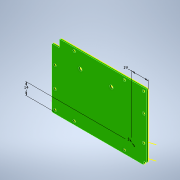
# Autodesk Inventor part: TCU_UCU_PCB
Saved by Autodesk Inventor 2021 (Build 250183000, 183)
## iProperties
Created: 2020-02-26
Part Number: TCU_UCU_PCB
Material: Generic
Document SubType Name: Modeling
Designer: lgnds
Density: 1 g/cm^3
Appearance: Default
Author: lgnds
Autodesk Inventor part; units mm, degrees
ref_plane "YZ Plane" through (0, 0, 0) normal (1, 0, 0) x (0, 1, 0)
ref_plane "XZ Plane" through (0, 0, 0) normal (0, 1, 0) x (-1, 0, 0)
ref_plane "XY Plane" through (0, 0, 0) normal (0, 0, 1) x (1, 0, 0)
sketch "Sketch1" plane through (0, 0, 0) normal (0, 0, 1) x (1, 0, 0)
  line L0 (-56.1965, -39.8485) -> (56.1965, -39.8485)
  line L1 (56.1965, -39.8485) -> (56.1965, 39.8485)
  line L2 (56.1965, 39.8485) -> (-56.1965, 39.8485)
  line L3 (-56.1965, 39.8485) -> (-56.1965, -39.8485)
  line L4 (-56.1965, -39.8485) -> (56.1965, 39.8485) construction
  line L5 (56.1965, -39.8485) -> (-56.1965, 39.8485) construction
  point P0 (0, 0)
  dimension "d0" = 79.697
  dimension "d1" = 112.393
  constraints: 12 end point, 2 midpoint, 2 parallel, 1 horizontal, 1 perpendicular
  measures "d0" distance of L2.end L0.start
  measures "d1" distance of L1.end L2.end
extrude "Extrusion1" add sketch "Sketch1" along normal blind 1.6
sketch "Sketch2" plane through (0, 0, 1.6) normal (0, 0, 1) x (1, 0, 0)
  line L0 (0, 0) -> (-76.7169, 0) construction
  line L1 (-76.7169, 0) -> (-68.8856, 0) construction
  line L2 (-56.1965, 39.8485) -> (-56.1965, -39.8485) construction
  circle A0 centre (-51.6965, 12.8485) radius 1.6
  line L3 (0, 55.7879) -> (0, -55.7879) construction
  line L4 (76.7169, 0) -> (68.8856, 0) construction
  line L5 (56.1965, 39.8485) -> (-56.1965, 39.8485) projected
  line L6 (-78.3509, -2) -> (74.4139, -2) construction
  line L7 (56.1965, 39.8485) -> (56.1965, -39.8485) construction
  circle A1 centre (51.6965, 12.8485) radius 1.6
  circle A2 centre (-51.6965, -16.8485) radius 1.6
  circle A3 centre (51.6965, -16.8485) radius 1.6
  dimension "d5" = 3.2
  dimension "d20" = 27
  dimension "d21" = 4.5
  dimension "d22" = 14.8485
  constraints: 10 end point, 6 symmetric about line, 4 centre point, 2 horizontal, 3 other
  measures "d5" diameter of A0
  measures "d20" distance from line of L5 A0.centre
  measures "d21" distance from line of L2 A0.centre
  measures "d22" distance from line of A0.centre L6
extrude "Extrusion2" cut sketch "Sketch2" against normal up to next
sketch "Sketch6" plane through (0, 0, 1.6) normal (0, 0, 1) x (1, 0, 0)
  line L0 (-64.772, 35.3485) -> (88.7849, 35.3485) construction
  circle A0 centre (-29.1965, 35.3485) radius 1.6
  line L1 (0, -55.7879) -> (0, 55.7879) construction
  line L2 (56.1965, 39.8485) -> (-56.1965, 39.8485) construction
  circle A1 centre (-51.6965, 12.8485) radius 1.6 projected
  line L3 (-95.4834, 0) -> (119.4963, 0) construction
  circle A2 centre (29.1965, 35.3485) radius 1.6
  circle A3 centre (-29.1965, -35.3485) radius 1.6
  circle A4 centre (29.1965, -35.3485) radius 1.6
  line L4 (-56.1965, 39.8485) -> (-56.1965, -39.8485) projected
  point P0 (0, 0)
  point P1 (-64.772, -35.3485)
  dimension "d23" = 3.2
  dimension "d24" = 4.5
  dimension "d36" = 27
  constraints: 4 centre point, 4 symmetric about line, 2 end point, 1 horizontal, 1 point on line, 3 other
  measures "d23" diameter of A0
  measures "d24" distance between parallel lines of L2 L0
  measures "d36" distance from line of L4 A0.centre
extrude "Extrusion5" cut sketch "Sketch6" against normal up to next contours A0 | A2 | A3 | A4
sketch "Sketch7" plane through (0, 0, 0) normal (0, 0, -1) x (-1, 0, 0)
  circle A0 centre (-14.1318, 20.7641) radius 1.9985
  arc A1 (51.6966, 24.8485) -> (51.6966, 14.8485) centre (51.6966, 19.8485) ccw
  line L0 (51.6966, 24.8485) -> (56.1965, 24.8485)
  line L1 (56.1965, 39.8485) -> (56.1965, -39.8485) construction
  line L2 (51.6966, 14.8485) -> (56.1965, 14.8485)
  line L3 (56.1965, 24.8485) -> (56.1965, 14.8485)
  circle A2 centre (22.0882, 20.7641) radius 1.9985
  line L4 (-91.8718, 0) -> (99.9198, 0) construction
  line L5 (-61.1962, -2.1515) -> (72.521, -2.1515) construction
  circle A3 centre (51.6966, -24.1515) radius 2 construction
  arc A4 (51.6966, -19.1515) -> (51.6966, -29.1515) centre (51.6966, -24.1515) ccw
  line L6 (51.6966, -29.1515) -> (56.1965, -29.1515)
  line L7 (56.1965, -44.1515) -> (56.1965, 35.5455) construction
  line L8 (51.6966, -19.1515) -> (56.1965, -19.1515)
  line L9 (56.1965, -29.1515) -> (56.1965, -19.1515)
  circle A5 centre (-14.1318, 20.7641) radius 1.4985 projected
  circle A6 centre (22.0882, 20.7641) radius 1.4985 projected
  circle A7 centre (51.6966, -24.1515) radius 2 projected
  circle A8 centre (51.6966, 19.8485) radius 2 projected
  point P0 (0, 0)
  dimension "d28" = 10
  dimension "d33" = 22
  constraints: 16 end point, 7 symmetric about line, 5 centre point, 4 point on circle, 4 point on line, 2 parallel, 2 tangent, 1 coincident, 1 horizontal, 2 other
  measures "d28" diameter of A1
  measures "d33" distance from line of A1.centre L5
extrude "Extrusion6" cut sketch "Sketch7" against normal up to next contours A0 | L0 L3 L2 A1 | A2 | L8 L9 L6 A4 | A5 | A6 | A7 | A8
thicken "Thicken1" operation add thickness 0.75 both sides no extend neighbours yes toward (-1, 0, 0) faces at (56.1965, -13.2828, 0.5333) (-18.7322, -39.8485, 0.5333) (-56.1965, -32.7172, 0.5333) (18.7322, 39.8485, 0.5333) (-56.1965, 34.8485, 0.5333)
thicken "Thicken2" operation add thickness 0.75 both sides no extend neighbours yes toward (1, 0, 0) faces at (-56.1965, 3.5152, 1.0667)
sketch "Sketch9" plane through (0, 0, 0) normal (0, 0, -1) x (-1, 0, 0)
  line L0 (-29.4046, -25) -> (-55.4465, -25)
  line L1 (-55.4465, -39.0985) -> (-55.4465, 39.0985) projected
  line L2 (55.4465, -39.0985) -> (-55.4465, -39.0985) projected
  line L3 (-42.5, -39.0985) -> (-42.5, -4.682)
  point P0 (0, 0)
  dimension "d43" = 42.5
  dimension "d44" = 25
  constraints: 4 end point, 2 point on line, 1 horizontal, 1 perpendicular
  measures "d43" distance from line of point (0, 0) L3
  measures "d44" distance from line of point (0, 0) L0
fillet "Fillet1" radius 1 6 edges at (-55.4465, -39.0985, 0.8) (-55.4465, -29.1515, 0.8) (-55.4465, -19.1515, 0.8) (55.4465, 39.0985, 0.8) (-55.4465, 24.8485, 0.8) (-55.4465, 14.8485, 0.8)
sketch "Sketch10" plane through (0, 0, 0) normal (0, 0, -1) x (-1, 0, 0)
  line L0 (55.4465, 39.0985) -> (46.4465, 39.0985)
  line L1 (46.4465, 39.0985) -> (46.4465, 30.0985)
  line L2 (46.4465, 30.0985) -> (55.4465, 30.0985)
  line L3 (55.4465, 30.0985) -> (55.4465, 39.0985)
  line L4 (-55.4465, -39.0985) -> (-55.4465, 38.0985) projected
  line L5 (-55.4465, -39.0985) -> (-51.6965, -39.0985)
  line L6 (-51.6965, -39.0985) -> (-51.6965, -35.3485)
  line L7 (-51.6965, -35.3485) -> (-55.4465, -35.3485)
  line L8 (-55.4465, -35.3485) -> (-55.4465, -39.0985)
  point P0 (0, 0)
  dimension "d48" = 9
  dimension "d49" = 9
  dimension "d72" = 3.75
  dimension "d73" = 3.75
  constraints: 16 end point, 4 parallel, 2 horizontal, 2 perpendicular
  measures "d48" distance of L0.end L1.end
  measures "d49" distance of L1.end L2.end
  measures "d72" distance of L5.end L6.end
  measures "d73" distance of L6.end L7.end
extrude "Extrusion7" cut sketch "Sketch10" against normal blind 10
fillet "Fillet3" radius 1 6 edges at (-46.4465, 39.0985, 0.8) (-46.4465, 30.0985, 0.8) (-55.4465, 30.0985, 0.8) (55.4465, -35.3485, 0.8) (51.6965, -35.3485, 0.8) (51.6965, -39.0985, 0.8)
sketch "Sketch11" plane through (0, 0, 0) normal (0, 0, -1) x (-1, 0, 0)
  circle A0 centre (-51.6965, 12.8485) radius 1.6 construction
  circle A1 centre (-29.1965, 35.3485) radius 1.6 construction
  line L0 (-51.6965, 12.8485) -> (-51.6965, 35.3485) construction
  circle A2 centre (-29.1965, 35.3485) radius 1.6 construction
  line L1 (-51.6965, 35.3485) -> (-29.1965, 35.3485) construction
  circle A3 centre (-51.6965, 35.3485) radius 1.6
  point P0 (0, 0)
  dimension "d53" = 3.2
  dimension "d54" = 3.2
  constraints: 4 end point, 1 centre point, 1 coincident, 1 perpendicular, 1 vertical
  measures "d53" diameter of A3
  measures "d54" diameter of A1
extrude "Extrusion8" cut sketch "Sketch11" against normal blind 10
sketch "Sketch12" plane through (0, 0, 0) normal (0, 0, -1) x (-1, 0, 0)
  circle A0 centre (51.6965, 12.8485) radius 1.6 projected
  circle A1 centre (51.6965, -16.8485) radius 1.6 projected
  point P0 (0, 0)
extrude "Extrusion9" add sketch "Sketch12" against normal up to surface (1.6 mm away)
sketch "Sketch13" plane through (0, 0, 0) normal (0, 0, -1) x (-1, 0, 0)
  line L0 (51.6965, 42.5451) -> (51.6965, -46.2521) construction
  line L1 (55.4465, 13.8485) -> (55.4465, -18.1515) projected
  circle A0 centre (29.1965, -35.3485) radius 1.6 projected
  line L2 (54.4465, -39.0985) -> (-50.6965, -39.0985) projected
  circle A1 centre (51.6965, 9.8485) radius 1.6
  circle A2 centre (51.6965, -14.1515) radius 1.6
  line L3 (54.4465, 30.0985) -> (47.4465, 30.0985) projected
  line L4 (-54.4465, 39.0985) -> (45.4465, 39.0985) projected
  line L5 (54.4465, 14.8485) -> (51.6966, 14.8485) projected
  line L6 (51.6966, -19.1515) -> (54.4465, -19.1515) projected
  point P0 (0, 0)
  point P1 (-49.5304, -39.0985)
  point P2 (-55.4465, -39.0985)
  point P3 (-51.6965, -39.0985)
  dimension "d61" = 3.75
  dimension "d62" = 3.75
  dimension "d63" = 3.2
  dimension "d64" = 3.2
  dimension "d65" = 3.2
  dimension "d67" = 29.25
  dimension "d68" = 5
  dimension "d69" = 5
  constraints: 2 centre point, 2 end point, 2 point on line, 1 vertical
  measures "d61" distance between parallel lines of L1 L0
  measures "d62" distance from line of L2 A0.centre
  measures "d63" diameter of A0
  measures "d64" diameter of A1
  measures "d65" diameter of A2
  measures "d67" distance from line of L4 A1.centre
  measures "d68" distance from line of L5 A1.centre
  measures "d69" distance from line of L6 A2.centre
extrude "Extrusion10" cut sketch "Sketch13" against normal blind 10 contours A1 | A2
sketch "Sketch14" plane through (0, 0, 0) normal (0, 0, -1) x (-1, 0, 0)
  circle A0 centre (29.1965, -35.3485) radius 1.6 construction
  circle A1 centre (51.6965, -14.1515) radius 1.6 construction
  circle A2 centre (29.1965, -35.3485) radius 1.6 construction
  line L0 (29.1965, -35.3485) -> (51.6965, -35.3485) construction
  line L1 (51.6965, -35.3485) -> (51.6965, -14.1515) construction
  circle A3 centre (51.6965, -35.3485) radius 1.6
  point P0 (0, 0)
  dimension "d74" = 3.2
  dimension "d75" = 3.2
  constraints: 4 end point, 1 centre point, 1 coincident, 1 horizontal, 1 perpendicular
  measures "d74" diameter of A1
  measures "d75" diameter of A3
extrude "Extrusion11" cut sketch "Sketch14" against normal up to next
sketch "Sketch18" plane through (0, 0, 0) normal (0, 0, -1) x (-1, 0, 0)
  line L0 (55.4465, 13.8485) -> (46.6966, 13.8485)
  line L1 (46.6966, 13.8485) -> (46.6966, 25.8485)
  line L2 (46.6966, 25.8485) -> (55.4465, 25.8485)
  line L3 (55.4465, 25.8485) -> (55.4465, 13.8485)
  line L4 (55.4465, -30.1515) -> (46.6966, -30.1515)
  line L5 (46.6966, -30.1515) -> (46.6966, -18.1515)
  line L6 (46.6966, -18.1515) -> (55.4465, -18.1515)
  line L7 (55.4465, -18.1515) -> (55.4465, -30.1515)
  arc A0 (51.6966, 24.8485) -> (51.6966, 14.8485) centre (51.6966, 19.8485) ccw projected
  arc A1 (51.6966, -19.1515) -> (51.6966, -29.1515) centre (51.6966, -24.1515) ccw projected
  point P0 (0, 0)
  constraints: 16 end point, 4 parallel, 2 horizontal, 2 perpendicular, 2 point on line, 2 tangent, 1 coincident
extrude "Extrusion12" add sketch "Sketch18" against normal up to surface (1.6 mm away)
sketch "CLIPS" plane through (0, 0, 0) normal (0, 0, -1) x (-1, 0, 0)
  line L0 (-36.4465, -29.7288) -> (-36.4465, -20.0562)
  line L1 (-36.4465, -25.0985) -> (-29.026, -25.0985)
  line L2 (-55.4465, -34.3485) -> (-55.4465, 38.0985) projected
  line L3 (54.4465, -39.0985) -> (-50.6965, -39.0985) projected
  circle A0 centre (-36.4465, -25.0985) radius 0.5
  point P0 (0, 0)
  dimension "d78" = 19
  dimension "d79" = 14
  dimension "d80" = 1
  constraints: 4 end point, 1 centre point, 1 coincident, 1 horizontal, 1 point on line, 1 vertical
  measures "d78" distance between parallel lines of L2 L0
  measures "d79" distance between parallel lines of L3 L1
  measures "d80" diameter of A0
sketch "OUTLINE" plane through (0, 0, 0) normal (0, 0, -1) x (-1, 0, 0)
  line L0 (-54.4465, 39.0985) -> (45.4465, 39.0985) projected
  arc A0 (-54.4465, 39.0985) -> (-55.4465, 38.0985) centre (-54.4465, 38.0985) ccw projected
  line L1 (-55.4465, -34.3485) -> (-55.4465, 38.0985) projected
  arc A1 (-55.4465, -34.3485) -> (-54.4465, -35.3485) centre (-54.4465, -34.3485) ccw projected
  line L2 (-54.4465, -35.3485) -> (-52.6965, -35.3485) projected
  arc A2 (-51.6965, -36.3485) -> (-52.6965, -35.3485) centre (-52.6965, -36.3485) ccw projected
  line L3 (-51.6965, -36.3485) -> (-51.6965, -38.0985) projected
  arc A3 (-51.6965, -38.0985) -> (-50.6965, -39.0985) centre (-50.6965, -38.0985) ccw projected
  line L4 (54.4465, -39.0985) -> (-50.6965, -39.0985) projected
  arc A4 (54.4465, -39.0985) -> (55.4465, -38.0985) centre (54.4465, -38.0985) ccw projected
  line L5 (55.4465, -30.1515) -> (55.4465, -38.0985) projected
  line L6 (55.4465, 13.8485) -> (55.4465, -18.1515) projected
  line L7 (55.4465, 29.0985) -> (55.4465, 25.8485) projected
  arc A5 (55.4465, 29.0985) -> (54.4465, 30.0985) centre (54.4465, 29.0985) ccw projected
  line L8 (54.4465, 30.0985) -> (47.4465, 30.0985) projected
  arc A6 (46.4465, 31.0985) -> (47.4465, 30.0985) centre (47.4465, 31.0985) ccw projected
  line L9 (46.4465, 31.0985) -> (46.4465, 38.0985) projected
  arc A7 (46.4465, 38.0985) -> (45.4465, 39.0985) centre (45.4465, 38.0985) ccw projected
  line L10 (55.4465, 13.8485) -> (55.4465, 25.8485)
  line L11 (55.4465, -30.1515) -> (55.4465, -18.1515)
  point P0 (0, 0)
  point P1 (55.4465, -29.9859)
  constraints: 4 end point, 1 collinear, 1 vertical
sketch "EXTRA" plane through (0, 0, 0) normal (0, 0, -1) x (-1, 0, 0)
  circle A0 centre (-29.1965, 35.3485) radius 1.6 projected
  circle A1 centre (-51.6965, 35.3485) radius 1.6 projected
  circle A2 centre (-51.6965, 12.8485) radius 1.6 projected
  circle A3 centre (-51.6965, -16.8485) radius 1.6 projected
  circle A4 centre (-29.1965, -35.3485) radius 1.6 projected
  circle A5 centre (29.1965, -35.3485) radius 1.6 projected
  circle A6 centre (51.6965, -14.1515) radius 1.6 projected
  circle A7 centre (22.0882, 20.7641) radius 1.9985 projected
  circle A8 centre (-14.1318, 20.7641) radius 1.9985 projected
  circle A9 centre (29.1965, 35.3485) radius 1.6 projected
  line L0 (-46.3087, -10.1785) -> (-47.3132, -12.4543) projected
  line L1 (-40.0751, -12.93) -> (-38.5846, -16.3071) projected
  line L2 (-46.4144, -16.3071) -> (-44.9239, -12.93) projected
  line L3 (-46.4995, -16.7109) -> (-46.4995, -17.7) projected
  line L4 (-38.4995, -17.7) -> (-38.4995, -16.7109) projected
  line L5 (-39.4411, -34.071) -> (-38.4366, -36.3468) projected
  line L6 (-38.5846, -33.6929) -> (-40.0751, -37.07) projected
  line L7 (-38.4995, -33.2891) -> (-38.4995, -32.3) projected
  line L8 (-44.9239, -37.07) -> (-46.4144, -33.6929) projected
  line L9 (-46.4995, -32.3) -> (-46.4995, -33.2891) projected
  line L10 (-47, -24.125) -> (-47, -25.875) projected
  line L11 (-37.973, -32.25) -> (-37.973, -17.75) projected
  line L12 (-64.473, -29.402) -> (-47.973, -33.25) projected
  line L13 (-47.973, -33.25) -> (-38.973, -33.25) projected
  line L14 (-38.973, -16.75) -> (-47.973, -16.75) projected
  line L15 (-47.973, -16.75) -> (-64.473, -12.902) projected
  line L16 (38.2302, -69.1917) -> (-30.2738, -69.1917) projected
  line L17 (38.2302, 29.4511) -> (-30.2738, 29.4511) projected
  line L18 (45.7992, -20.1299) -> (45.7992, 21.8821) projected
  line L19 (-30.2738, -27.6989) -> (38.2302, -27.6989) projected
  line L20 (-37.8428, 21.8821) -> (-37.8428, -20.1299) projected
  line L21 (6.0102, -13.4274) -> (32.8067, -13.4274) projected
  line L22 (-24.8503, -13.4274) -> (1.9462, -13.4274) projected
  circle A10 centre (51.6966, -35.348) radius 1.5 projected
  circle A11 centre (-43.9995, -19) radius 0.49 projected
  circle A12 centre (51.6966, 9.8485) radius 1.5 projected
  arc A13 (-40.0751, -12.93) -> (-44.9239, -12.93) centre (-42.4995, -14) ccw projected
  arc A14 (-38.4995, -16.7109) -> (-38.5846, -16.3071) centre (-39.4995, -16.7109) ccw projected
  circle A15 centre (-40.9995, -31) radius 0.49 projected
  arc A16 (-46.4144, -16.3071) -> (-46.4995, -16.7109) centre (-45.4995, -16.7109) ccw projected
  arc A17 (-38.5846, -33.6929) -> (-38.4995, -33.2891) centre (-39.4995, -33.2891) ccw projected
  arc A18 (-44.9239, -37.07) -> (-40.0751, -37.07) centre (-42.4995, -36) ccw projected
  arc A19 (-46.4995, -33.2891) -> (-46.4144, -33.6929) centre (-45.4995, -33.2891) ccw projected
  arc A20 (-38.973, -33.25) -> (-37.973, -32.25) centre (-38.973, -32.25) ccw projected
  arc A21 (-37.973, -17.75) -> (-38.973, -16.75) centre (-38.973, -17.75) ccw projected
  circle A22 centre (-22.9728, 9.7171) radius 0.4955 projected
  circle A23 centre (30.9272, -7.9629) radius 0.4955 projected
  circle A24 centre (-5.2928, -7.9629) radius 0.4955 projected
  circle A25 centre (13.2472, 9.7171) radius 0.4955 projected
  arc A26 (45.7992, 21.8821) -> (38.2302, 29.4511) centre (38.2302, 21.8821) ccw projected
  arc A27 (38.2302, -27.6989) -> (45.7992, -20.1299) centre (38.2302, -20.1299) ccw projected
  arc A28 (-37.8428, -20.1299) -> (-30.2738, -27.6989) centre (-30.2738, -20.1299) ccw projected
  arc A29 (-30.2738, 29.4511) -> (-37.8428, 21.8821) centre (-30.2738, 21.8821) ccw projected
  arc A30 (-30.1685, -16.3342) -> (-27.3083, -17.7661) centre (-30.2863, -20.1424) ccw projected
  arc A31 (2.3753, -16.686) -> (5.5824, -16.6866) centre (3.9782, -20.1424) ccw projected
  arc A32 (35.2646, -17.7661) -> (38.1248, -16.3342) centre (38.2427, -20.1424) ccw projected
  point P0 (0, 0)
  constraints: 1 horizontal alignment, 2 other
equation "\"d33\" = 0.5 * d32"
equation "\"d49\" = d48"
equation "\"d73\" = d72"
equation "\"d53\" = d54"
equation "\"d64\" = d63"
equation "\"d65\" = d63"
equation "\"d69\" = d68"
equation "\"d75\" = d74"
equation "\"d31\" = d30"
equation "\"d32\" = 44"
equation "\"d30\" = 0.5"
body "Solid1"
